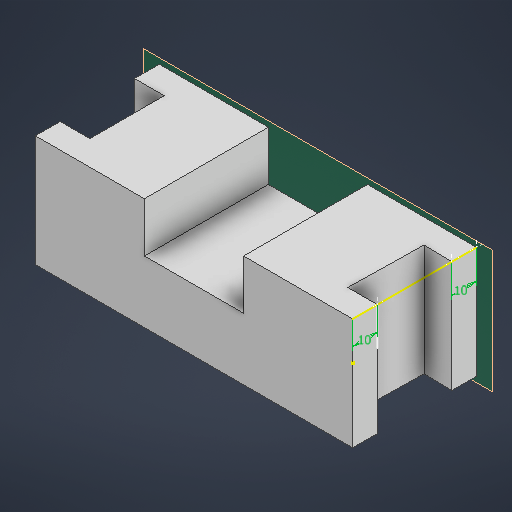
# Autodesk Inventor part: Part10
Saved by Autodesk Inventor 2026.2 (Build 302298000, 298)
## iProperties
Created: 2026-05-04
Part Number: Part10
Material: Generic
Document SubType Name: Modeling
Designer: LENOVO
Density: 1 g/cm^3
Appearance: Default
Author: LENOVO
Autodesk Inventor part; units mm, degrees
ref_plane "YZ Plane" through (0, 0, 0) normal (1, 0, 0) x (0, 1, 0)
ref_plane "XZ Plane" through (0, 0, 0) normal (0, 1, 0) x (-1, 0, 0)
ref_plane "XY Plane" through (0, 0, 0) normal (0, 0, 1) x (1, 0, 0)
sketch "Sketch1" plane through (0, 0, 0) normal (0, 0, 1) x (1, 0, 0)
  line L0 (-52.1514, 15.2486) -> (75.8486, 15.2486)
  line L1 (75.8486, 15.2486) -> (75.8486, -29.7514)
  line L2 (75.8486, -29.7514) -> (-52.1514, -29.7514)
  line L3 (-52.1514, -29.7514) -> (-52.1514, 15.2486)
  point P0 (0, 0)
  dimension "d0" = 128
  dimension "d1" = 128
  dimension "d2" = 45
  constraints: 8 end point, 2 perpendicular, 1 horizontal
  measures "d0" distance of L0.start L0.end
  measures "d1" distance of L1.end L2.end
  measures "d2" distance of L0.end L1.end
extrude "Extrusion1" add sketch "Sketch1" against normal blind 50
ref_plane "Work Plane1" through (0, 0, -50) normal (0, 0, -1) x (-1, 0, 0)
sketch "Sketch2" plane through (0, 0, -50) normal (0, 0, -1) x (-1, 0, 0)
  line L0 (52.1514, 15.2486) -> (-75.8486, 15.2486) projected
  line L1 (-31.8486, 15.2486) -> (-31.8486, -4.7514)
  line L2 (-31.8486, -4.7514) -> (8.1514, -4.7514)
  line L3 (8.1514, -4.7514) -> (8.1514, 15.2486)
  point P0 (0, 0)
  dimension "d6" = 44
  dimension "d7" = 44
  dimension "d8" = 20
  constraints: 6 end point, 2 perpendicular, 2 point on line, 1 coincident, 1 vertical
  measures "d6" distance of point (52.151, 15.249) L3.end
  measures "d7" distance of L0.end L1.start
  measures "d8" distance of L2.end L3.end
extrude "Extrusion2" cut sketch "Sketch2" against normal blind 50
sketch "Sketch3" plane through (75.8486, -29.7514, 0) normal (1, 0, 0) x (0, 0, -1)
  line L0 (0, 45) -> (50, 45) projected
  line L1 (10, 45) -> (10, 29.7514)
  point P0 (0, 29.7514)
  point P1 (40, 45)
  dimension "d11" = 10
  dimension "d12" = 10
  constraints: 2 end point, 2 point on line, 1 coincident, 1 vertical
  measures "d11" distance of L0.start L1.start
  measures "d12" distance of point (50, 45) point (40, 45)
sketch "Sketch4" plane through (75.8486, 15.2486, 0) normal (0, 1, 0) x (1, 0, 0)
  line L0 (0, 0) -> (0, 50) projected
  line L1 (0, 50) -> (-128, 50) projected
  line L2 (0, 10) -> (-12, 10)
  line L3 (-12, 10) -> (-11.4432, 40.2365)
  line L4 (-11.4432, 40.2365) -> (0.5568, 40.0155)
  point P0 (-75.8486, 0)
  point P1 (0, 40.0258)
  dimension "d13" = 10
  dimension "d14" = 10
  dimension "d15" = 12
  dimension "d16" = 12
  constraints: 6 end point, 2 coincident, 1 horizontal, 1 perpendicular, 1 point on line
  measures "d13" distance of L0.start L2.start
  measures "d14" distance of point (0, 50) L4.end
  measures "d15" distance of L2.start L2.end
  measures "d16" horizontal distance of L3.end L4.end
extrude "Extrusion3" cut sketch "Sketch4" against normal blind 50
sketch "Sketch5" plane through (31.8486, 15.2486, 0) normal (0, 1, 0) x (1, 0, 0)
  line L0 (-84, 0) -> (-84, 50) projected
  line L1 (44, 50) -> (-84, 50) projected
  line L2 (-84, 10) -> (-72, 10)
  line L3 (-72, 10) -> (-72, 40)
  line L4 (-72, 40) -> (-84, 40)
  point P0 (-31.8486, 0)
  dimension "d19" = 10
  dimension "d20" = 10
  dimension "d21" = 12
  dimension "d22" = 12
  constraints: 6 end point, 2 perpendicular, 1 coincident, 1 horizontal, 1 point on line
  measures "d19" distance of L0.start L2.start
  measures "d20" distance of point (-84, 50) L4.end
  measures "d21" distance of L2.start L2.end
  measures "d22" distance of L3.end L4.end
extrude "Extrusion4" cut sketch "Sketch5" against normal blind 50
body "Solid1"
